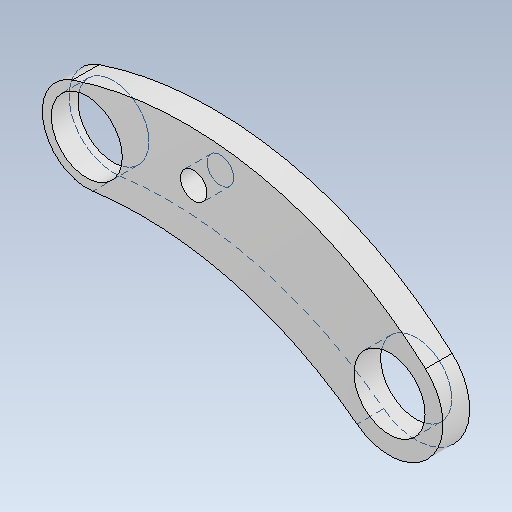
# Autodesk Inventor part: heikousita
Saved by Autodesk Inventor 2020 (Build 240168000, 168)
## iProperties
Created: 2021-02-23
Part Number: heikousita
Material: アルミニウム 2014-T4
Document SubType Name: Modeling
Designer: AA19065
Density: 2.8 g/cm^3
Appearance: サテン
Mass: 3.52665 g
Surface Area: 13.4064 cm^2
Volume: 1.25952 cm^3
Author: AA19065
Autodesk Inventor part; units mm, degrees
ref_plane "YZ Plane" through (0, 0, 0) normal (1, 0, 0) x (0, 1, 0)
ref_plane "XZ Plane" through (0, 0, 0) normal (0, 1, 0) x (-1, 0, 0)
ref_plane "XY Plane" through (0, 0, 0) normal (0, 0, 1) x (1, 0, 0)
sketch "スケッチ1" plane through (0, 0, 0) normal (0, 0, 1) x (1, 0, 0)
  circle A0 centre (104.0735, 2) radius 6.025
  arc A1 (100.4168, -2.7885) -> (70.6822, 5.0468) centre (76.1402, -34.5791) ccw
  line L0 (69.7806, -5) -> (104.0735, 2) construction
  circle A2 centre (69.7806, -5) radius 5 construction
  arc A3 (102.7574, -3.8795) -> (72.4739, -9.2126) centre (94.0202, -42.9136) ccw construction
  circle A4 centre (75.3506, 22) radius 5 construction
  circle A5 centre (70, 10) radius 1.5
  circle A6 centre (70, 10) radius 5
  arc A7 (109.4834, 4.652) -> (75.6055, 26.9935) centre (73.5667, -12.9545) ccw construction
  arc A8 (108.1244, 6.4599) -> (68.3957, 14.7356) centre (81.2303, -23.1494) ccw
  arc A9 (105.8851, 7.7462) -> (66.341, -1.371) centre (93.8576, -30.4027) ccw construction
  line L1 (70, 10) -> (104.0735, 2) construction
  circle A10 centre (82.0403, 11.2819) radius 1.5
  line L2 (48.483, 55.1333) -> (82.5564, 47.1333) construction
  line L3 (82.5564, 47.1333) -> (53.8336, 67.1333) construction
  line L4 (82.5564, 47.1333) -> (48.2636, 40.1333) construction
  circle A11 centre (53.8336, 67.1333) radius 5 construction
  circle A12 centre (48.2636, 40.1333) radius 5 construction
  circle A13 centre (48.483, 55.1333) radius 5
  circle A14 centre (82.5564, 47.1333) radius 1.5
  circle A15 centre (82.5564, 47.1333) radius 5
  circle A16 centre (48.483, 55.1333) radius 1.5
  arc A17 (77.6092, 46.4087) -> (54.8703, 62.242) centre (58.8098, 43.6549) ccw construction
  arc A18 (78.225, 44.6356) -> (51.2502, 50.9689) centre (61.7656, 35.1441) ccw
  arc A19 (79.6686, 43.0516) -> (52.5201, 37.51) centre (68.6948, 27.5411) ccw construction
  arc A20 (85.2716, 51.3319) -> (44.1201, 42.9319) centre (68.9807, 26.1405) ccw construction
  arc A21 (86.7799, 49.8095) -> (45.8918, 59.4095) centre (61.4389, 33.7524) ccw
  arc A22 (87.4691, 48.0636) -> (53.0017, 72.0636) centre (57.993, 42.4818) ccw construction
  circle A23 centre (82.5564, 47.1333) radius 4
  circle A24 centre (104.0735, 2) radius 4
  circle A25 centre (70, 10) radius 4
  point P0 (0, 0)
  point P1 (0, 0)
  point P2 (0, 0)
  dimension "d0" = 40
  dimension "d1" = 10
  dimension "d2" = 40
  dimension "d3" = 10
  dimension "d4" = 10
  dimension "d5" = 3
  dimension "d6" = 19
  dimension "d7" = 30
  dimension "d8" = 3
  dimension "d9" = 8
  dimension "d10" = 8
  dimension "d11" = 8
  constraints: 43 point on circle, 25 centre point, 21 tangent, 12 coincident, 10 end point, 10 equal radius, 15 other
  measures "d0" radius of A1
  measures "d1" diameter of A6
  measures "d2" radius of A8
  measures "d3" diameter of A15
  measures "d4" diameter of A13
  measures "d5" diameter of A16
  measures "d6" radius of A18
  measures "d7" radius of A21
  measures "d8" diameter of A14
  measures "d9" diameter of A23
  measures "d10" diameter of A24
  measures "d11" diameter of A25
extrude "押し出し1" add sketch "スケッチ1" along normal blind 3 contours A0 | A0 A1 A6 A8 | A6
